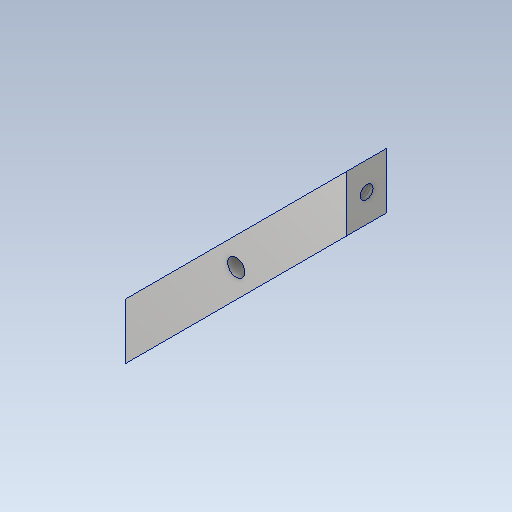
# Autodesk Inventor part: FAB-OX0026-CameraSupportCrossBrace
Saved by Autodesk Inventor 2020 (Build 240168000, 168)
## iProperties
Created: 2017-02-27
Part Number: FAB-OX0026-CameraSupportCrossBrace
Material: Aluminum 6061
Document SubType Name: Modeling
Designer: map
Density: 2.7 g/cm^3
Appearance: Aluminum - Flat
Mass: 65.6699 g
Surface Area: 80.8338 cm^2
Volume: 24.3222 cm^3
Author: map
Autodesk Inventor part; units mm, degrees
ref_plane "YZ Plane" through (0, 0, 0) normal (1, 0, 0) x (0, 1, 0)
ref_plane "XZ Plane" through (0, 0, 0) normal (0, 1, 0) x (-1, 0, 0)
ref_plane "XY Plane" through (0, 0, 0) normal (0, 0, 1) x (1, 0, 0)
sketch "Sketch1" plane through (0, 0, 0) normal (0, 0, 1) x (1, 0, 0)
  line L0 (-42, -52.6066) -> (42, 31.3934)
  line L1 (42, 52.6066) -> (-42, -31.3934)
  line L2 (-42, -52.6066) -> (42, 52.6066) construction
  line L3 (42, 31.3934) -> (-42, -31.3934) construction
  line L4 (-42, -52.6066) -> (93.2082, -52.6066) construction
  line L5 (42, 52.6066) -> (42, 31.3934)
  line L6 (-42, -31.3934) -> (-42, -52.6066)
  point P0 (0, 0)
  point P1 (0, 0)
  dimension "d0" = 45
  dimension "d2" = 15
  dimension "d38" = 84
  constraints: 14 end point, 3 midpoint, 2 parallel, 1 coincident, 1 horizontal
  measures "d0" angle of L4 L0
  measures "d2" distance between parallel lines of L1 L0
  measures "d38" distance between parallel lines of L5 L6
extrude "Extrusion1" add sketch "Sketch1" along normal blind 15
sketch "Sketch2" plane through (0, 0, 0) normal (0, 0, -1) x (-1, 0, 0)
  line L0 (42, -52.6066) -> (-42, 31.3934) construction
  line L1 (42, -31.3934) -> (42, -52.6066) construction
  line L2 (-42, 52.6066) -> (42, -31.3934) construction
  line L3 (-42, 31.3934) -> (-42, 52.6066) construction
  line L4 (-10.6066, 0) -> (0, 10.6066)
  line L5 (0, 10.6066) -> (10.6066, 0)
  line L6 (10.6066, 0) -> (0, -10.6066)
  line L7 (0, -10.6066) -> (-10.6066, 0)
  line L8 (-10.6066, 0) -> (10.6066, 0) construction
  line L9 (0, 10.6066) -> (0, -10.6066) construction
  line L10 (-42, 52.6066) -> (42, -31.3934) projected
  line L11 (-42, 52.6066) -> (42, -52.6066) construction
  line L12 (42, -52.6066) -> (-42, 31.3934) construction
  point P0 (0, 0)
  point P1 (0, 0)
  dimension "d5" = 15
  dimension "d7" = 15
  constraints: 14 end point, 4 midpoint, 2 parallel, 2 perpendicular, 2 point on line
  measures "d5" distance of L4.start L4.end
  measures "d7" distance of L4.end L5.end
extrude "Extrusion2" cut sketch "Sketch2" against normal blind 7.5
hole "CentralM6Clearance" at (0, 0, 0) direction (0, 0, 1) diameter 6.6 end through all clearance for "Socket Head Cap Screw ISO 4762" size "M6" standard "ISO"
sketch "Sketch4" plane through (-42, -52.6066, 0) normal (-1, 0, 0) x (0, 0, 1)
  line L0 (0, 0) -> (0, 21.2132) construction
  line L1 (0, 21.2132) -> (15, 21.2132) construction
  line L2 (15, 21.2132) -> (15, 0) construction
  line L3 (15, 0) -> (0, 0) construction
  line L4 (0, 21.2132) -> (15, 0) construction
  line L5 (0, 21.2132) -> (15, 21.2132) construction
  line L6 (0, 0) -> (15, 0) construction
  line L7 (15, 21.2132) -> (0, 0) construction
  point P0 (0, 52.6066)
  point P1 (7.5, 10.6066)
  constraints: 4 end point, 1 midpoint
hole "M6Tap1" at (-42, -42, 7.5) direction (1, 0, 0) diameter 4.917 depth 12 tip angle 118 thread size "M6x1" class "6H" standard "ISO Metric profile"
sketch "Sketch5" plane through (42, 31.3934, 0) normal (1, 0, 0) x (0, 0, -1)
  line L0 (0, 21.2132) -> (0, 0) projected
  line L1 (0, 0) -> (-15, 0) projected
  line L2 (-15, 0) -> (-15, 21.2132) projected
  line L3 (-15, 21.2132) -> (0, 21.2132) projected
  line L4 (0, 0) -> (-15, 0) projected
  line L5 (-15, 21.2132) -> (0, 0)
  point P0 (-7.5, 10.6066)
  constraints: 2 end point, 1 midpoint
hole "Hole3" at (42, 42, 7.5) direction (-1, 0, 0) diameter 4.917 depth 12 tip angle 118 thread size "M6x1" class "6H" standard "ISO Metric profile"
derived "FAB-P0042 - Camera Bracket sCMOS.ipt"
equation "\"d3\" = d2"
equation "\"d5\" = d2"
equation "\"d8\" = 0.5 * d2"
body "Solid1"
